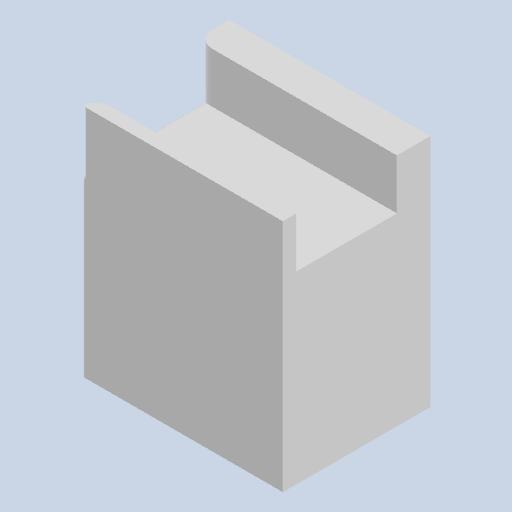
# Autodesk Inventor part: upor2
Saved by Autodesk Inventor 2022 (Build 260153000, 153)
## iProperties
Created: 2024-12-11
Part Number: upor2
Material: Типовые
Document SubType Name: Modeling
Designer: Andrey
Density: 1 g/cm^3
Appearance: По умолчанию
Author: Andrey
Autodesk Inventor part; units mm, degrees
ref_plane "YZ Plane" through (0, 0, 0) normal (1, 0, 0) x (0, 1, 0)
ref_plane "XZ Plane" through (0, 0, 0) normal (0, 1, 0) x (-1, 0, 0)
ref_plane "XY Plane" through (0, 0, 0) normal (0, 0, 1) x (1, 0, 0)
sketch "Эскиз1" plane through (0, 0, 0) normal (0, 0, 1) x (1, 0, 0)
  line L0 (-0.9994, -4.532) -> (-0.9994, -7) projected
  line L1 (-0.9994, -7) -> (4.0006, -7) projected
  line L2 (4.0006, -7) -> (4.0006, 7) projected
  line L3 (4.0006, 7) -> (1.6539, 7) projected
  arc A0 (1.6539, 7) -> (-1.5392, 5.8477) centre (1.6539, 2) ccw projected
  spline S0 degree 3 poles (-1.5392, 5.8477) (-1.841, 5.5961) (-2.3851, 5.1007) (-2.9171, 4.5079) (-3.3417, 3.9411) (-3.598, 3.5113) (-3.8018, 3.0569) (-3.8945, 2.7699) (-3.9568, 2.4926) (-3.9838, 2.3119) (-4.0006, 2.0887) (-4.0006, 1.9113) (-3.9838, 1.6881) (-3.9568, 1.5074) (-3.8945, 1.2301) (-3.8018, 0.9431) (-3.598, 0.4887) (-3.3417, 0.0589) (-2.9342, -0.485) (-2.6405, -0.8158) (-2.428, -1.0328) knots -1 -1 -1 -1 -0.916667 -0.833333 -0.791667 -0.708333 -0.666667 -0.604167 -0.583333 -0.541667 -0.520833 -0.479167 -0.458333 -0.416667 -0.395833 -0.333333 -0.291667 -0.208333 -0.166667 -0.091743 -0.091743 -0.091743 -0.091743 projected
  spline S1 degree 3 poles (-2.428, -1.0328) (-2.2019, -1.2635) (-1.7947, -1.7688) (-1.3413, -2.6303) (-1.0622, -3.563) (-0.9994, -4.209) (-0.9994, -4.532) knots -1 -1 -1 -1 -0.75 -0.5 -0.25 0 0 0 0 projected
  circle A1 centre (28.5006, -1) radius 2.1 projected
  circle A2 centre (-2.1462, 18.5) radius 2.1 projected
  circle A3 centre (-9.0714, -1) radius 2.1 projected
  spline S2 degree 3 poles (-2.4745, 7.8043) (-2.4902, 7.5514) (-2.5538, 7.3036) (-2.7702, 6.8452) (-2.921, 6.6386) (-3.1063, 6.4657) knots 0 0 0 0 0.076038 0.076038 0.152076 0.152076 0.152076 0.152076 projected
  arc A4 (-2.2745, 9.4079) -> (-2.4745, 7.8043) centre (10.5006, 7) ccw projected
  line L4 (8.0006, -7) -> (40.3538, -7) projected
  line L5 (40.3538, -7) -> (22.9061, 16.2926) projected
  arc A5 (22.9061, 16.2926) -> (10.5006, 22.5) centre (10.5006, 7) ccw projected
  line L6 (10.5006, 22.5) -> (-10.3517, 22.5) projected
  line L7 (-10.3517, 22.5) -> (-11.2994, 21.5522) projected
  arc A6 (-11.2994, 21.5522) -> (-11.8548, 20.4853) centre (-9.8852, 20.138) ccw projected
  line L8 (-11.8548, 20.4853) -> (-11.9558, 19.9127) projected
  line L9 (-11.9558, 19.9127) -> (-6.1462, 19.9127) projected
  line L10 (-6.1462, 19.9127) -> (-6.1462, 17.7127) projected
  line L11 (-6.1462, 17.7127) -> (-12.3437, 17.7127) projected
  line L12 (-12.3437, 17.7127) -> (-16.3486, -5) projected
  line L13 (-16.3486, -5) -> (-9.5088, -5) projected
  line L14 (-9.5088, -5) -> (-9.5088, -7) projected
  line L15 (-9.5088, -7) -> (-2.4994, -7) projected
  line L16 (-2.4994, -7) -> (-2.4994, -3.9012) projected
  spline S3 degree 3 poles (-3.1312, -2.4424) (-2.9413, -2.6206) (-2.7879, -2.8341) (-2.6206, -3.201) (-2.5754, -3.3369) (-2.5147, -3.616) (-2.4994, -3.7584) (-2.4994, -3.9012) knots 0 0 0 0 0.078129 0.078129 0.12097 0.12097 0.16381 0.16381 0.16381 0.16381 projected
  spline S4 degree 2 poles (-3.1312, -2.4424) (-7.8801, 2.0117) (-3.1063, 6.4657) knots -0.944242 -0.944242 -0.944242 -0.053426 -0.053426 -0.053426 projected
  line L17 (23.5006, -7) -> (11.5006, -7)
  line L18 (11.5006, -7) -> (11.5006, 7)
  line L19 (11.5006, 7) -> (23.5006, 7)
  line L20 (23.5006, -7) -> (23.5006, 7)
  spline S5 degree 3 poles (-1.1225, 10.2083) (-1.2509, 10.2303) (-1.3823, 10.2271) (-1.6365, 10.1704) (-1.7568, 10.1175) (-1.9705, 9.9686) (-2.0617, 9.874) (-2.2023, 9.656) (-2.2506, 9.5349) (-2.2745, 9.4079) knots 0 0 0 0 0.039064 0.039064 0.078129 0.078129 0.117193 0.117193 0.155946 0.155946 0.155946 0.155946 projected
  spline S6 degree 2 poles (-1.1225, 10.2083) (8.092, 8.6257) (8.0006, 7) knots 0.047114 0.047114 0.047114 1 1 1 projected
  line L21 (8.0006, 7) -> (8.0006, -7) projected
  point P0 (0, 0)
  dimension "d0" = 12
  constraints: 8 end point, 2 perpendicular, 1 horizontal, 1 point on circle
  measures "d0" distance of L17.start L17.end
extrude "Выдавливание1" add sketch "Эскиз1" against normal blind 10 contours L18 L19 L20 L4
sketch "Эскиз2" plane through (11.5006, -7, 0) normal (-1, 0, 0) x (0, 0, 1)
  line L0 (0, 14) -> (0, 0) projected
  line L1 (0, 14) -> (-10, 14) projected
  line L2 (-10, 0) -> (-10, 14) projected
  line L3 (0, 0) -> (-10, 0) projected
  line L4 (0, 14) -> (-10, 14) projected
  line L5 (-5, 14) -> (-5, 0)
  circle A0 centre (-5, 7) radius 2.1
  point P0 (0, 7)
  dimension "d3" = 4.2
  constraints: 3 midpoint, 2 end point, 1 centre point
  measures "d3" diameter of A0
extrude "Выдавливание2" cut sketch "Эскиз2" against normal blind 11 contours A0 L5 | L5 A0
sketch "Эскиз3" plane through (11.5006, -7, 0) normal (-1, 0, 0) x (0, 0, 1)
  circle A0 centre (-5, 7) radius 2.1 projected
  line L0 (0, 14) -> (0, 0) projected
  line L1 (0, 14) -> (-10, 14) projected
  line L2 (-10, 0) -> (-10, 14) projected
  line L3 (0, 0) -> (-10, 0) projected
  line L4 (0, 14) -> (-10, 14) projected
  line L5 (-2, 14) -> (-8, 14)
  line L6 (-8, 14) -> (-8, 11)
  line L7 (-8, 11) -> (-2, 11)
  line L8 (-2, 11) -> (-2, 14)
  point P0 (0, 7)
  dimension "d6" = 2
  dimension "d7" = 2
  dimension "d8" = 3
  constraints: 8 end point, 2 parallel, 1 horizontal, 1 perpendicular, 1 point on line
  measures "d6" distance between parallel lines of L2 L6
  measures "d7" distance between parallel lines of L0 L8
  measures "d8" distance between parallel lines of L1 L7
extrude "Выдавливание3" cut sketch "Эскиз3" against normal blind 15 contours L8 L7 L6 L1
fillet "Сопряжение1" radius 1 3 edges at (11.5006, 5.5, -8) (11.5006, 4, -5) (11.5006, 5.5, -2)
sketch "Эскиз4" plane through (0, 0, 0) normal (0, 0, 1) x (1, 0, 0)
  line L0 (11.5006, 7) -> (11.5006, -7) projected
  line L1 (23.5006, 7) -> (11.5006, 7) projected
  line L2 (23.5006, -7) -> (23.5006, 7) projected
  line L3 (8.0006, -7) -> (40.3538, -7) projected
  point P0 (0, 0)
extrude "Выдавливание4" cut sketch "Эскиз4" against normal blind 1.2
fillet "Сопряжение2" radius 0.2 3 edges at (11.5056, 3.1005, -1.2) (11.5006, -2, -1.2) (11.5208, 5.1, -1.2)
